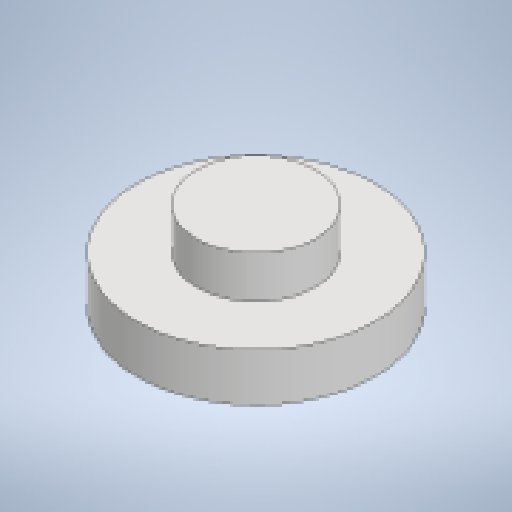
# Autodesk Inventor part: base
Saved by Autodesk Inventor 2025.4 (Build 294407000, 407)
## iProperties
Created: 2026-03-19
Part Number: base
Material: Generic
Document SubType Name: Modeling
Designer: dawid
Density: 1 g/cm^3
Appearance: Default
Author: dawid
Autodesk Inventor part; units mm, degrees
ref_plane "YZ Plane" through (0, 0, 0) normal (1, 0, 0) x (0, 1, 0)
ref_plane "XZ Plane" through (0, 0, 0) normal (0, 1, 0) x (-1, 0, 0)
ref_plane "XY Plane" through (0, 0, 0) normal (0, 0, 1) x (1, 0, 0)
sketch "Sketch1" plane through (0, 0, 0) normal (0, 0, 1) x (1, 0, 0)
  line L0 (0, 0) -> (0, 150)
  line L1 (0, 150) -> (100, 150)
  line L2 (100, 150) -> (100, 80)
  line L3 (100, 80) -> (200, 80)
  line L4 (200, 80) -> (200, 0)
  line L5 (0, 0) -> (200, 0)
  dimension "d0" = 150
  dimension "d1" = 100
  dimension "d2" = 90
  dimension "d3" = 70
  dimension "d4" = 100
  constraints: 12 end point, 4 perpendicular, 1 horizontal, 1 vertical
  measures "d0" distance of L0.start L0.end
  measures "d1" distance of L0.end L1.end
  measures "d2" angle of L0 L1
  measures "d3" distance of L1.end L2.end
  measures "d4" distance of L2.end L3.end
revolve "Revolution1" add sketch "Sketch1" angle 360 about axis through (0, 0, 0) along (0, 1, 0)
body "Solid1"
